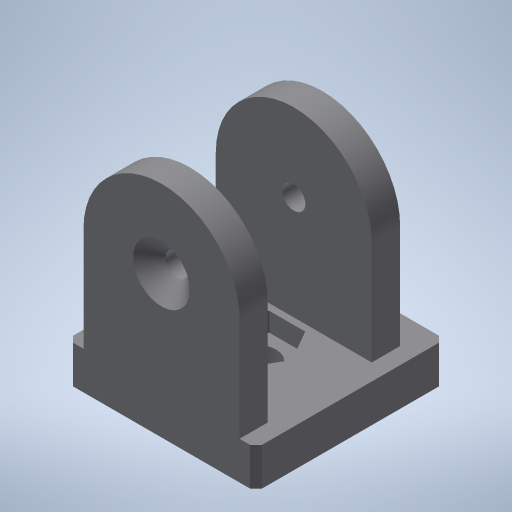
# Autodesk Inventor part: Robotunits GUS_4040 75
Saved by Autodesk Inventor 2023 (Build 270158000, 158)
## iProperties
Created: 2023-08-22
Part Number: Robotunits GUS_4040 75
Material: Generic
Catalog Web Link: www.cadenas.de
Description: GUS 4040-Elbow
Vendor: ROBOTUNITS
Document SubType Name: Modeling
Designer: psAdmin
Manufacturer: ROBOTUNITS
Mass: 21.6736 g
Surface Area: 114.75 cm^2
Volume: 21.6736 cm^3
Density: 1 g/cm^3
Appearance: PSOLRGB-175-175-175
Category: PARTsolutions
Company: ROBOTUNITS
PSOL_IDENT_0: {$CADENAS_DATA/23d-libs/robotunits/profil_und_verbindungstechnik/verbindungstechnik_raster_40/parts/
PSOL_IDENT_1: gus_4_41.prj},195 {VTYP=3D},{NB=Robotunits GUS_4040 75},{LINA=Robotunits GUS_4040},{NN=GUS 4040},{DA
PSOL_IDENT_2: TE=01.02.2021 09:12:11},{GEOMDATE=05.01.2012 16:03:00},{VERSION=},{LINEID=10},{WBVAR=WINKEL},{WBNUME
PSOL_IDENT_3: RIC=WINKEL}  {NB=Robotunits GUS_4040 75},{LINA=Robotunits GUS_4040},{KT=DUMMY},{ARTIKEL=GUS_4040},{W
PSOL_IDENT_4: INKEL=75},{FORM=1.000}
NB: Robotunits GUS_4040 75
NN: GUS 4040
NT: Elbow
NBSYN: Robotunits $ARTIKEL. $WINKEL.
LINA: Robotunits GUS_4040
CATALOG: Robotunits
ARTIKEL: GUS_4040
WINKEL: 75
FORM: 1
SUPPLIER: ROBOTUNITS
ARTICLENO: Robotunits GUS_4040 75
BOMINFO: Robotunits GUS_4040
CREATOR: CADENAS GmbH
Title: Robotunits GUS_4040
Author: Cadenas PARTsolutions
Comments: Elbow
Autodesk Inventor part; units mm, degrees
ref_plane "YZ Plane" through (0, 0, 0) normal (1, 0, 0) x (0, 1, 0)
ref_plane "XZ Plane" through (0, 0, 0) normal (0, 1, 0) x (-1, 0, 0)
ref_plane "XY Plane" through (0, 0, 0) normal (0, 0, 1) x (1, 0, 0)
sketch "Skizze_1" plane through (0, 0, 0) normal (0, 1, 0) x (-1, 0, 0)
  line L0 (20, -20) -> (20, 20)
  line L1 (20, 20) -> (-20, 20)
  line L2 (-20, 20) -> (-20, -20)
  line L3 (-20, -20) -> (20, -20)
  constraints: 8 end point
extrude "Extrusion1" add sketch "Skizze_1" along normal blind 52
sketch "Skizze_2" plane through (0, 0, 0) normal (1, 0, 0) x (0, 1, 0)
  line L0 (55, 20) -> (46.5, 20)
  line L1 (46.5, 20) -> (46.5, 14)
  line L2 (46.5, 14) -> (8, 14)
  line L3 (8, 14) -> (8, -8)
  line L4 (8, -8) -> (46.5, -8)
  line L5 (46.5, -8) -> (46.5, -14)
  line L6 (46.5, -14) -> (8, -14)
  line L7 (8, -14) -> (8, -20)
  line L8 (8, -20) -> (55, -20)
  line L9 (55, -20) -> (55, 20)
  constraints: 20 end point
extrude "Extrusion2" cut sketch "Skizze_2" along normal mid plane 42
sketch "Skizze_3" plane through (0, 0, 0) normal (0, 0, 1) x (1, 0, 0)
  line L0 (-20, 53) -> (-20, 8)
  line L1 (-20, 8) -> (-16.5, 8)
  line L2 (-16.5, 8) -> (-16.5, 30)
  arc A0 (16.5, 30) -> (-16.5, 30) centre (0, 30) ccw
  line L3 (16.5, 30) -> (16.5, 8)
  line L4 (16.5, 8) -> (20, 8)
  line L5 (20, 8) -> (20, 53)
  line L6 (20, 53) -> (-20, 53)
  constraints: 14 end point, 2 point on circle, 1 centre point
extrude "Extrusion3" cut sketch "Skizze_3" along normal mid plane 42
sketch "Sketch4" plane through (-20, 0, 20) normal (0, 0, 1) x (1, 0, 0)
  point P0 (20, 30)
hole "Hole1" at (0, 30, 20) direction (0, 0, -1) diameter 4.92 depth 39.8 countersink diameter 12 countersink angle 94.019
sketch "Sketch_1" plane through (0, 0, 0) normal (0, 1, 0) x (-1, 0, 0)
  line L0 (9.025, -10.45) -> (-9.025, -10.45)
  line L1 (-9.025, -10.45) -> (-9.025, -18.5)
  line L2 (-9.025, -18.5) -> (9.025, -18.5)
  line L3 (9.025, -18.5) -> (9.025, -10.45)
  constraints: 8 end point
extrude "Extrusion4" cut sketch "Sketch_1" along normal blind 6.5
sketch "Sketch_2" plane through (0, 0, 0) normal (0, 1, 0) x (-1, 0, 0)
  line L0 (9.025, 10.45) -> (9.025, 18.5)
  line L1 (9.025, 18.5) -> (-9.025, 18.5)
  line L2 (-9.025, 18.5) -> (-9.025, 10.45)
  line L3 (-9.025, 10.45) -> (9.025, 10.45)
  constraints: 8 end point
extrude "Extrusion5" cut sketch "Sketch_2" along normal blind 6.5
sketch "Sketch_3" plane through (0, 0, 0) normal (0, 1, 0) x (-1, 0, 0)
  line L0 (-10.45, 9.025) -> (-18.5, 9.025)
  line L1 (-18.5, 9.025) -> (-18.5, -9.025)
  line L2 (-18.5, -9.025) -> (-10.45, -9.025)
  line L3 (-10.45, -9.025) -> (-10.45, 9.025)
  constraints: 8 end point
extrude "Extrusion6" cut sketch "Sketch_3" along normal blind 6.5
sketch "Sketch_4" plane through (0, 0, 0) normal (0, 1, 0) x (-1, 0, 0)
  line L0 (18.5, 9.025) -> (10.45, 9.025)
  line L1 (10.45, 9.025) -> (10.45, -9.025)
  line L2 (10.45, -9.025) -> (18.5, -9.025)
  line L3 (18.5, -9.025) -> (18.5, 9.025)
  constraints: 8 end point
extrude "Extrusion7" cut sketch "Sketch_4" along normal blind 6.5
sketch "Sketch9" plane through (0, 0, 0) normal (0, -1, 0) x (1, 0, 0)
  point P0 (0, 0)
hole "Hole2" at (0, 0, 0) direction (0, 1, 0) diameter 8.5 depth 8
sketch "Sketch_5" plane through (0, 8, 0) normal (0, 1, 0) x (1, 0, 0)
  line L0 (-7.621, 0) -> (-3.8105, -6.6)
  line L1 (-3.8105, -6.6) -> (3.8105, -6.6)
  line L2 (3.8105, -6.6) -> (7.621, 0)
  line L3 (7.621, 0) -> (3.8105, 6.6)
  line L4 (3.8105, 6.6) -> (-3.8105, 6.6)
  line L5 (-3.8105, 6.6) -> (-7.621, 0)
  constraints: 12 end point
extrude "Extrusion8" cut sketch "Sketch_5" against normal blind 4
ref_plane "GN300Klemmhebel_XY" through (0, 29.8, 20) normal (0, 0, 1) x (1, 0, 0)
ref_plane "GN300Klemmhebel_YZ" through (0, 29.8, 20) normal (1, 0, 0) x (0, 1, 0)
ref_plane "GN300Klemmhebel_ZX" through (0, 29.8, 20) normal (0, 1, 0) x (0, 0, 1)
ref_plane "GUS_4_41_XY" through (0, 29.8, 0) normal (0, 0, 1) x (1, 0, 0)
ref_plane "GUS_4_41_YZ" through (0, 29.8, 0) normal (1, 0, 0) x (0, 1, 0)
ref_plane "GUS_4_41_ZX" through (0, 29.8, 0) normal (0, 1, 0) x (0, 0, 1)
ref_plane "GUS_4_41_L_XY" through (0, 29.8, -20) normal (0, 0, 1) x (1, 0, 0)
ref_plane "GUS_4_41_L_YZ" through (0, 29.8, -20) normal (1, 0, 0) x (0, 1, 0)
ref_plane "GUS_4_41_L_ZX" through (0, 29.8, -20) normal (0, 1, 0) x (0, 0, 1)
ref_plane "GUS_4_41_R_XY" through (0, 29.8, 20) normal (0, 0, 1) x (1, 0, 0)
ref_plane "GUS_4_41_R_YZ" through (0, 29.8, 20) normal (1, 0, 0) x (0, 1, 0)
ref_plane "GUS_4_41_R_ZX" through (0, 29.8, 20) normal (0, 1, 0) x (0, 0, 1)
ref_plane "p0_XY" through (0, 0, 0) normal (0, 1, 0) x (1, 0, 0)
ref_plane "p0_YZ" through (0, 0, 0) normal (1, 0, 0) x (0, 0, -1)
ref_plane "p0_ZX" through (0, 0, 0) normal (0, 0, -1) x (0, 1, 0)
ref_plane "p1_XY" through (0, 0, -14.475) normal (0, 1, 0) x (1, 0, 0)
ref_plane "p1_YZ" through (0, 0, -14.475) normal (1, 0, 0) x (0, 0, -1)
ref_plane "p1_ZX" through (0, 0, -14.475) normal (0, 0, -1) x (0, 1, 0)
ref_plane "p2_XY" through (14.475, 0, 0) normal (0, 1, 0) x (1, 0, 0)
ref_plane "p2_YZ" through (14.475, 0, 0) normal (1, 0, 0) x (0, 0, -1)
ref_plane "p2_ZX" through (14.475, 0, 0) normal (0, 0, -1) x (0, 1, 0)
ref_plane "p3_XY" through (0, 0, 14.475) normal (0, 1, 0) x (1, 0, 0)
ref_plane "p3_YZ" through (0, 0, 14.475) normal (1, 0, 0) x (0, 0, -1)
ref_plane "p3_ZX" through (0, 0, 14.475) normal (0, 0, -1) x (0, 1, 0)
ref_plane "p4_XY" through (-14.475, 0, 0) normal (0, 1, 0) x (1, 0, 0)
ref_plane "p4_YZ" through (-14.475, 0, 0) normal (1, 0, 0) x (0, 0, -1)
ref_plane "p4_ZX" through (-14.475, 0, 0) normal (0, 0, -1) x (0, 1, 0)
ref_plane "ps_XY" through (0, 8, 0) normal (0, 1, 0) x (1, 0, 0)
ref_plane "ps_YZ" through (0, 8, 0) normal (1, 0, 0) x (0, 0, -1)
ref_plane "ps_ZX" through (0, 8, 0) normal (0, 0, -1) x (0, 1, 0)
chamfer "Chamfer1" distance 1.25 angle 45 4 edges at (-20, 4, 20) (20, 4, 20) (-20, 4, -20) (20, 4, -20)
body "Solid1"
